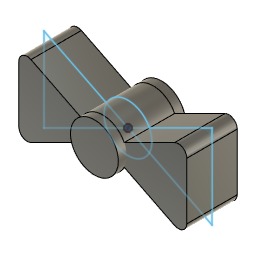
smart walking cane (Autodesk Fusion 360 archive; units mm, degrees)
design "switch"
Autodesk Fusion 360 part; units mm, degrees
sketch "Sketch1" plane through (0, 0, 0) normal (0, 1, 0) x (1, 0, 0)
  circle A0 centre (0, 0) radius 14.2396
  line L0 (0, 0) -> (50, -25)
  line L1 (50, -25) -> (50, 25)
  line L2 (50, 25) -> (0, 0)
  line L3 (0, 0) -> (-50, -25)
  line L4 (-50, -25) -> (-50, 25)
  line L5 (-50, 25) -> (0, 0)
  constraint coincident A0.centre L0.start
  constraint vertical L1
  constraint parallel L2 L3
  constraint parallel L1 L4
  constraint parallel L0 L5
extrude "Extrude1" add sketch "Sketch1" along normal mid plane 40 contours A0 L0 L2 | A0 L2 L5 | A0 L0 L3 | A0 L3 L5 makes body 1
extrude "Extrude2" add sketch "Sketch1" along normal mid plane 30 separate body makes body 2
fillet "Fillet1" radius 5 4 edges at (50, 0, 25) (50, 0, -25) (-50, 0, 25) (-50, 0, -25) on bodies 2

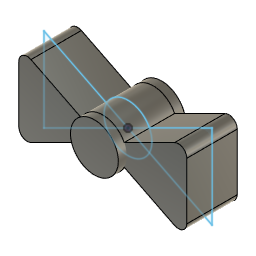
design "switch"
Autodesk Fusion 360 part; units mm, degrees
sketch "Sketch1" plane through (0, 0, 0) normal (0, 1, 0) x (1, 0, 0)
  circle A0 centre (0, 0) radius 14.2396
  line L0 (0, 0) -> (50, -25)
  line L1 (50, -25) -> (50, 25)
  line L2 (50, 25) -> (0, 0)
  line L3 (0, 0) -> (-50, -25)
  line L4 (-50, -25) -> (-50, 25)
  line L5 (-50, 25) -> (0, 0)
  constraint coincident A0.centre L0.start
  constraint vertical L1
  constraint parallel L2 L3
  constraint parallel L1 L4
  constraint parallel L0 L5
extrude "Extrude1" add sketch "Sketch1" along normal mid plane 40 contours A0 L0 L2 | A0 L2 L5 | A0 L0 L3 | A0 L3 L5 makes body 1
extrude "Extrude2" add sketch "Sketch1" along normal mid plane 30 separate body makes body 2
fillet "Fillet1" radius 5 4 edges at (50, 0, 25) (50, 0, -25) (-50, 0, 25) (-50, 0, -25) on bodies 2

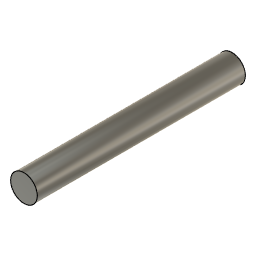
design "pipe"
Autodesk Fusion 360 part; units mm, degrees
sketch "Sketch1" plane through (0, 0, 0) normal (0, 1, 0) x (1, 0, 0)
  circle A0 centre (0, 0) radius 45
  dimension "d1" = 90
  constraint coincident A0.centre origin
  measures "d1" diameter of A0
extrude "Extrude1" add sketch "Sketch1" along normal blind 700

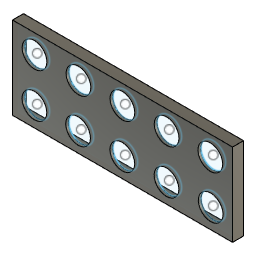
design "aluminium box"
Autodesk Fusion 360 part; units mm, degrees
sketch "Sketch1" plane through (0, 0, 0) normal (0, 1, 0) x (1, 0, 0)
  line L0 (-50, -25) -> (50, -25)
  line L1 (50, -25) -> (50, 25)
  line L2 (50, 25) -> (-50, 25)
  line L3 (-50, 25) -> (-50, -25)
  line L4 (-45, -20) -> (-45, 20)
  line L5 (-45, 20) -> (45, 20)
  line L6 (45, 20) -> (45, -20)
  line L7 (45, -20) -> (-45, -20)
  constraint horizontal L0
  constraint perpendicular L0 L1
  constraint perpendicular L1 L2
  constraint perpendicular L0 L3
  constraint perpendicular L0 L4
  constraint perpendicular L3 L5
  constraint perpendicular L5 L6
  constraint perpendicular L4 L7
extrude "Extrude1" add sketch "Sketch1" along normal blind 2 contours L4 L5 L6 L7
sketch "Sketch2" plane through (0, 0, 0) normal (0, 1, 0) x (1, 0, 0)
  line L0 (40, 15) -> (-40, 15)
  line L1 (-40, 15) -> (-40, -15)
  line L2 (-40, -15) -> (40, -15)
  line L3 (40, -15) -> (40, 15)
  constraint horizontal L0
  constraint perpendicular L0 L1
  constraint perpendicular L1 L2
  constraint perpendicular L0 L3
extrude "Extrude2" add sketch "Sketch2" against normal blind 2
extrude "Extrude3" cut 1 faces at (13.3333, 0, 18.3333) along direction (0, 1, 0) blind 2
sketch "Sketch3" plane through (0, 2, 0) normal (0, 1, 0) x (-1, 0, 0)
  line L0 (40, -15) -> (40, 15)
  line L1 (40, 15) -> (-40, 15)
  line L2 (-40, 15) -> (-40, -15)
  line L3 (-40, -15) -> (40, -15)
  line L4 (39, -14) -> (39, 14)
  line L5 (39, 14) -> (-39, 14)
  line L6 (-39, 14) -> (-39, -14)
  line L7 (-39, -14) -> (39, -14)
  constraint vertical L4
  constraint perpendicular L4 L5
  constraint perpendicular L5 L6
  constraint perpendicular L4 L7
extrude "Extrude4" cut sketch "Sketch3" against normal blind 3 contours L4 L5 L6 L7
sketch "Sketch4" plane through (0, -1, 0) normal (0, 1, 0) x (-1, 0, 0)
  line L0 (-39, -14) -> (39, -14)
  line L1 (39, -14) -> (39, 14)
  line L2 (39, 14) -> (-39, 14)
  line L3 (-39, 14) -> (-39, -14)
  circle A0 centre (32, 8) radius 4.5
  circle A1 centre (16, 8) radius 4.5
  circle A2 centre (0, 8) radius 4.5
  circle A3 centre (-16, 8) radius 4.5
  circle A4 centre (-32, 8) radius 4.5
  circle A5 centre (32, -8) radius 4.5
  circle A6 centre (16, -8) radius 4.5
  circle A7 centre (0, -8) radius 4.5
  circle A8 centre (-16, -8) radius 4.5
  circle A9 centre (-32, -8) radius 4.5
  dimension "d9" = 9
  dimension "d12" = -64
  dimension "d13" = 0
  dimension "d14" = 7
  measures "d9" diameter of A0
  measures "d14" distance of L1 A0.centre
hole "Hole1" at (16.0386, -2, 8.0304) direction (0, 1, 0) diameter 9 depth 4 tip angle 180
hole "Hole2" at (31.9264, 0, 7.7981) direction (0, -1, 0) diameter 9 depth 4 tip angle 180
hole "Hole3" at (-0.0476, -1, 8.0158) direction (0, -1, 0) diameter 9 depth 4 tip angle 180
hole "Hole4" at (-16.0135, -1, 7.9487) direction (0, -1, 0) diameter 9 depth 4 tip angle 180
hole "Hole5" at (-31.9977, -1, 8.0302) direction (0, -1, 0) diameter 9 depth 4 tip angle 180
hole "Hole6" at (32.0607, -1, -7.9452) direction (0, -1, 0) diameter 9 depth 4 tip angle 180
hole "Hole7" at (15.9921, -1, -8.0674) direction (0, -1, 0) diameter 9 depth 4 tip angle 180
hole "Hole8" at (-0.0765, -1, -8.0674) direction (0, -1, 0) diameter 9 depth 4 tip angle 180
hole "Hole9" at (-16.1451, -1, -8.0063) direction (0, -1, 0) diameter 9 depth 4 tip angle 180
hole "Hole10" at (-32.0377, -1, -7.9439) direction (0, -1, 0) diameter 9 depth 4 tip angle 180
